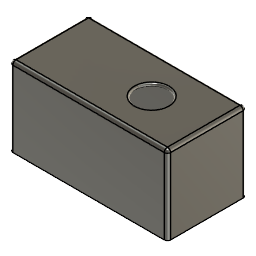
Throttle Box Assembly (Autodesk Fusion 360 archive; units mm, degrees)
design "Cover"
part number: 2026-03-17-12-51-27-306
Autodesk Fusion 360 part; units mm, degrees
sketch "Bottom" plane through (0, 0, 0) normal (0, 0, 1) x (1, 0, 0)
  line L0 (48, 25) -> (-48, 25)
  line L1 (-50, 23) -> (-50, -23)
  line L2 (-48, -25) -> (48, -25)
  line L3 (50, -23) -> (50, 23)
  line L4 (50, 25) -> (-50, -25) construction
  line L5 (-50, 25) -> (50, -25) construction
  arc A0 (-48, 25) -> (-50, 23) centre (-48, 23) ccw
  arc A1 (-50, -23) -> (-48, -25) centre (-48, -23) ccw
  arc A2 (48, -25) -> (50, -23) centre (48, -23) ccw
  arc A3 (50, 23) -> (48, 25) centre (48, 23) ccw
  line L6 (-50, 25) -> (-47, 25)
  line L7 (-47, 25) -> (-47, 22)
  line L8 (-47, 22) -> (-50, 22)
  line L9 (-50, 22) -> (-50, 25)
  circle A4 centre (-47, 22) radius 1.75
  circle A5 centre (-47, 22) radius 3
  line L10 (48, -23) -> (48, 23)
  line L11 (48, 23) -> (-48, 23)
  line L12 (-48, 23) -> (-48, -23)
  line L13 (-48, -23) -> (48, -23)
  circle A6 centre (47, 22) radius 3
  circle A7 centre (47, 22) radius 1.75
  circle A8 centre (-47, -22) radius 3
  circle A9 centre (-47, -22) radius 1.75
  circle A10 centre (47, -22) radius 3
  circle A11 centre (47, -22) radius 1.75
  dimension "d1" = 100
  dimension "d2" = 50
  dimension "d3" = 2
  dimension "d5" = 3
  dimension "d6" = 3
  dimension "d7" = 3.5
  dimension "d8" = 6
  dimension "d23" = -2
  dimension "d62" = 94
  dimension "d63" = -44
  constraint horizontal L0
  constraint perpendicular L0 L1
  constraint parallel L0 L2
  constraint parallel L1 L3
  constraint coincident L4 origin
  constraint coincident L5 origin
  constraint coincident L5.start L0
  constraint coincident L5.start L1
  constraint tangent L0 A0
  constraint tangent L1 A0
  constraint coincident L4.end L1
  constraint coincident L4.end L2
  constraint tangent L1 A1
  constraint tangent L2 A1
  constraint equal A0 A1
  constraint coincident L5.end L2
  constraint coincident L5.end L3
  constraint tangent L2 A2
  constraint tangent L3 A2
  constraint equal A0 A2
  constraint coincident L4.start L3
  constraint coincident L4.start L0
  constraint tangent L3 A3
  constraint tangent L0 A3
  constraint equal A0 A3
  constraint horizontal L6
  constraint vertical L7
  constraint horizontal L8
  constraint vertical L9
  constraint coincident L7.end L8.start
  constraint concentric A4 A5
  measures "d1" distance of L4.end L5.end
  measures "d2" distance of L5.start L4.end
  measures "d3" radius of A0
  measures "d5" distance of L5.start L6.end
  measures "d6" distance of L5.start L8.end
  measures "d7" diameter of A4
  measures "d8" diameter of A5
extrude "Extrude3" add sketch "Bottom" along normal blind 48 contours L0 L1 A0 L6 L9 A5 | L7 A4 A5 L11 | L7 L8 A4 A5 | L0 A5 L11 A6 | L0 L3 A3 A6 | L10 L11 A6 A7 | L1 A5 L12 A8 | L8 A4 A5 L12 | A4 A5 L11 L12 | L3 L10 A6 A10 | L10 L11 A6 A7 | L1 L2 A1 A8 | L12 L13 A8 A9 | L10 L13 A10 A11 | L2 L3 A2 A10 | L12 L13 A8 A9 | L2 L13 A8 A10 | L10 L13 A10 A11
sketch "Top" plane through (0, 0, 48) normal (0, 0, 1) x (-1, 0, 0)
  circle A0 centre (47, 22) radius 1.75
  circle A1 centre (-47, -22) radius 1.75
  circle A2 centre (-47, 22) radius 1.75
  line L0 (48, 19.1716) -> (48, -19.1716)
  arc A3 (48, -19.1716) -> (44.1716, -23) centre (47, -22) ccw
  line L1 (44.1716, -23) -> (-44.1716, -23)
  arc A4 (-44.1716, -23) -> (-48, -19.1716) centre (-47, -22) ccw
  line L2 (-48, -19.1716) -> (-48, 19.1716)
  arc A5 (-48, 19.1716) -> (-44.1716, 23) centre (-47, 22) ccw
  line L3 (-44.1716, 23) -> (44.1716, 23)
  arc A6 (44.1716, 23) -> (48, 19.1716) centre (47, 22) ccw
  circle A7 centre (47, -22) radius 1.75
  arc A8 (50, 23) -> (48, 25) centre (48, 23) ccw
  line L4 (48, 25) -> (-48, 25)
  arc A9 (-48, 25) -> (-50, 23) centre (-48, 23) ccw
  line L5 (-50, 23) -> (-50, -23)
  arc A10 (-50, -23) -> (-48, -25) centre (-48, -23) ccw
  line L6 (-48, -25) -> (48, -25)
  arc A11 (48, -25) -> (50, -23) centre (48, -23) ccw
  line L7 (50, -23) -> (50, 23)
  line L8 (-45, -20) -> (15, -20)
  line L9 (15, -20) -> (15, 20)
  line L10 (15, 20) -> (-45, 20)
  line L11 (-45, 20) -> (-45, -20)
  line L12 (20, -15.6) -> (45, -15.6)
  line L13 (45, -15.6) -> (45, 15.6)
  line L14 (45, 15.6) -> (20, 15.6)
  line L15 (20, 15.6) -> (20, -15.6)
  line L16 (20, -15.6) -> (45, 15.6) construction
  line L17 (45, -15.6) -> (20, 15.6) construction
  line L18 (43, 13.6) -> (22, 13.6)
  line L19 (22, 13.6) -> (22, -13.6)
  line L20 (22, -13.6) -> (43, -13.6)
  line L21 (43, -13.6) -> (43, 13.6)
  circle A12 centre (-15, 0) radius 10
  line L22 (30, -10.6) -> (35, -10.6)
  line L23 (35, -10.6) -> (35, -5.6)
  line L24 (35, -5.6) -> (30, -5.6)
  line L25 (30, -5.6) -> (30, -10.6)
  point P0 (32.5, 0)
  dimension "d68" = 60
  dimension "d69" = 40
  dimension "d70" = 25
  dimension "d71" = 31.2
  dimension "d72" = -2
  dimension "d73" = 20
  dimension "d77" = 5
  dimension "d78" = 5
  constraint horizontal L8
  constraint vertical L9
  constraint horizontal L10
  constraint vertical L11
  constraint horizontal L12
  constraint perpendicular L12 L13
  constraint parallel L12 L14
  constraint parallel L13 L15
  constraint coincident L16 P0
  constraint coincident L17 P0
  constraint horizontal L22
  constraint vertical L23
  constraint horizontal L24
  constraint vertical L25
  measures "d68" distance of L8.start L8.end
  measures "d69" distance of L8.start L10.end
  measures "d70" distance of L13.end L14.end
  measures "d71" distance of L12.end L13.end
  measures "d73" diameter of A12
  measures "d77" distance of L22.start L22.end
  measures "d78" distance of L22.start L24.end
extrude "Extrude8" add sketch "Top" along normal blind 2 contours A0 | A1 | A2 | L0 A3 L1 A4 A5 L3 A6 L8 L9 L10 | A4 A5 L8 L9 L10 L11 | A5 L10 L11 | A4 L8 L11 | A4 L2 A5 L11 | A7 | A8 L4 A9 L5 A10 L6 A11 L7 | L12 L13 L14 L15 | L18 L19 L20 L21 | A12 | L22 L23 L24 L25
fillet "Fillet13" radius 2 8 edges at (50, 0, 50) (49.4142, 24.4142, 50) (0, 25, 50) (-49.4142, 24.4142, 50) (-50, 0, 50) (-49.4142, -24.4142, 50) (0, -25, 50) (49.4142, -24.4142, 50)
extrude "Extrude9" cut sketch "Top" along normal blind 2 contours A12
extrude "Extrude10" add sketch "Top" against normal blind 11.5 contours L22 L23 L24 L25
fillet "Fillet14" radius 2 8 edges at (-30, 8.1, 48) (-30, 5.6, 42.25) (-30, 10.6, 42.25) (-35, 10.6, 42.25) (-35, 5.6, 42.25) (-32.5, 5.6, 48) (-35, 8.1, 48) (-32.5, 10.6, 48)
fillet "Fillet15" radius 1 2 edges at (24.3233, 3.6162, 48) (24.3233, -3.6162, 50)
fillet "Fillet16" radius 1 16 edges at (44.1716, -23, 24) (48, -19.1716, 24) (48, 19.1716, 24) (44.1716, 23, 24) (-44.1716, 23, 24) (-48, 19.1716, 24) (-48, -19.1716, 24) (-44.1716, -23, 24) (-48, 0, 48) (-44.8787, -19.8787, 48) (0, -23, 48) (44.8787, -19.8787, 48) (48, 0, 48) (0, 23, 48) (44.8787, 19.8787, 48) (-44.8787, 19.8787, 48)
equation "d51 = 'Control ESP32: WYGB, WYG, WG, B Curtis: RYBG Bypass: YW F/R: YG, BW'"

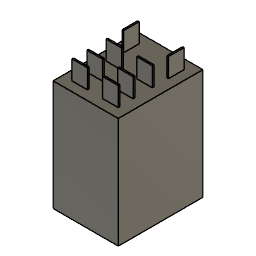
design "YJ2N-LY 24VDC Relay"
part number: 2026-03-24-09-30-35-597
Autodesk Fusion 360 part; units mm, degrees
sketch "Bottom" plane through (0, 0, 0) normal (0, 0, 1) x (1, 0, 0)
  line L0 (10.4, 13.5) -> (-10.4, 13.5)
  line L1 (-10.4, 13.5) -> (-10.4, -13.5)
  line L2 (-10.4, -13.5) -> (10.4, -13.5)
  line L3 (10.4, -13.5) -> (10.4, 13.5)
  line L4 (10.4, 13.5) -> (-10.4, -13.5) construction
  line L5 (-10.4, 13.5) -> (10.4, -13.5) construction
  dimension "d1" = 20.8
  dimension "d2" = 27
  constraint horizontal L0
  constraint perpendicular L0 L1
  constraint parallel L0 L2
  constraint parallel L1 L3
  constraint coincident L4 origin
  constraint coincident L5 origin
  measures "d1" distance of L1.end L2.end
  measures "d2" distance of L0.end L1.end
extrude "Extrude1" add sketch "Bottom" along normal blind 35.25
sketch "Top" plane through (0, 0, 35.25) normal (0, 0, 1) x (-1, 0, 0)
  line L0 (-10.4, 13.5) -> (-10.4, -13.5)
  line L1 (-10.4, -13.5) -> (10.4, -13.5)
  line L2 (10.4, -13.5) -> (10.4, 13.5)
  line L3 (10.4, 13.5) -> (-10.4, 13.5)
  line L4 (-7.4, -10.5) -> (-6.9, -10.5)
  line L5 (-6.9, -10.5) -> (-6.9, -5.5)
  line L6 (-6.9, -5.5) -> (-7.4, -5.5)
  line L7 (-7.4, -5.5) -> (-7.4, -10.5)
  line L8 (6.9, -5.5) -> (6.9, -10.5)
  line L9 (6.9, -10.5) -> (7.4, -10.5)
  line L10 (7.4, -10.5) -> (7.4, -5.5)
  line L11 (7.4, -5.5) -> (6.9, -5.5)
  line L12 (7.4, 10.5) -> (2.4, 10.5)
  line L13 (2.4, 10.5) -> (2.4, 10)
  line L14 (2.4, 10) -> (7.4, 10)
  line L15 (7.4, 10) -> (7.4, 10.5)
  line L16 (-7.4, 10.5) -> (-7.4, 10)
  line L17 (-7.4, 10) -> (-2.4, 10)
  line L18 (-2.4, 10.5) -> (-7.4, 10.5)
  line L19 (-2.4, 10) -> (-2.4, 10.5)
  line L20 (2.4, 5.7) -> (2.4, 5.2)
  line L21 (2.4, 5.2) -> (7.4, 5.2)
  line L22 (7.4, 5.7) -> (2.4, 5.7)
  line L23 (7.4, 5.2) -> (7.4, 5.7)
  line L24 (-7.4, 5.7) -> (-7.4, 5.2)
  line L25 (-7.4, 5.2) -> (-2.4, 5.2)
  line L26 (-2.4, 5.7) -> (-7.4, 5.7)
  line L27 (-2.4, 5.2) -> (-2.4, 5.7)
  line L28 (-7.4, -0.9) -> (-2.4, -0.9)
  line L29 (-7.4, -0.4) -> (-7.4, -0.9)
  line L30 (-2.4, -0.9) -> (-2.4, -0.4)
  line L31 (2.4, -0.4) -> (2.4, -0.9)
  line L32 (2.4, -0.9) -> (7.4, -0.9)
  line L33 (7.4, -0.4) -> (2.4, -0.4)
  line L34 (-2.4, -0.4) -> (-7.4, -0.4)
  line L35 (7.4, -0.9) -> (7.4, -0.4)
  dimension "d7" = 0.5
  dimension "d8" = 5
  dimension "d11" = 14.3
  dimension "d12" = 0
  dimension "d15" = 5
  dimension "d16" = 0.5
  dimension "d19" = -9.8
  dimension "d20" = -4.8
  dimension "d23" = 0
  dimension "d24" = -6.1
  constraint horizontal L4
  constraint vertical L5
  constraint horizontal L6
  constraint vertical L7
  constraint horizontal L12
  constraint vertical L13
  constraint horizontal L14
  constraint vertical L15
  measures "d7" distance of L4.start L4.end
  measures "d8" distance of L4.start L6.end
  measures "d15" distance of L12.start L12.end
  measures "d16" distance of L12.start L14.end
extrude "Extrude2" add sketch "Top" along normal blind 6.1 contours L4 L5 L6 L7 | L8 L9 L10 L11 | L12 L13 L14 L15 | L16 L17 L18 L19 | L20 L21 L22 L23 | L24 L25 L26 L27 | L28 L29 L30 L34 | L31 L32 L33 L35

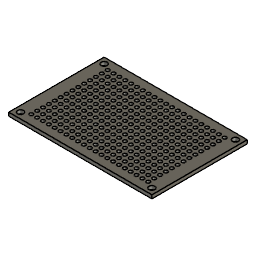
design "Perfboard"
part number: 2026-02-25-23-39-29-210
Autodesk Fusion 360 part; units mm, degrees
sketch "Bottom" plane through (0, 0, 0) normal (0, 0, 1) x (1, 0, 0)
  line L0 (30, 20) -> (-30, 20)
  line L1 (-30, 20) -> (-30, -20)
  line L2 (-30, -20) -> (30, -20)
  line L3 (30, -20) -> (30, 20)
  line L4 (30, 20) -> (-30, -20) construction
  line L5 (-30, 20) -> (30, -20) construction
  circle A0 centre (-27.5, 17.5) radius 1.25
  circle A1 centre (27.5, 17.5) radius 1.25
  circle A2 centre (-27.5, -17.5) radius 1.25
  circle A3 centre (27.5, -17.5) radius 1.25
  circle A4 centre (-24.5, 16) radius 0.75
  circle A5 centre (-22.05, 16) radius 0.75
  circle A6 centre (-19.6, 16) radius 0.75
  circle A7 centre (-17.15, 16) radius 0.75
  circle A8 centre (-14.7, 16) radius 0.75
  circle A9 centre (-12.25, 16) radius 0.75
  circle A10 centre (-9.8, 16) radius 0.75
  circle A11 centre (-7.35, 16) radius 0.75
  circle A12 centre (-4.9, 16) radius 0.75
  circle A13 centre (-2.45, 16) radius 0.75
  circle A14 centre (0, 16) radius 0.75
  circle A15 centre (2.45, 16) radius 0.75
  circle A16 centre (4.9, 16) radius 0.75
  circle A17 centre (7.35, 16) radius 0.75
  circle A18 centre (9.8, 16) radius 0.75
  circle A19 centre (12.25, 16) radius 0.75
  circle A20 centre (14.7, 16) radius 0.75
  circle A21 centre (17.15, 16) radius 0.75
  circle A22 centre (19.6, 16) radius 0.75
  circle A23 centre (22.05, 16) radius 0.75
  circle A24 centre (24.5, 16) radius 0.75
  circle A25 centre (-24.5, 13.5385) radius 0.75
  circle A26 centre (-22.05, 13.5385) radius 0.75
  circle A27 centre (-19.6, 13.5385) radius 0.75
  circle A28 centre (-17.15, 13.5385) radius 0.75
  circle A29 centre (-14.7, 13.5385) radius 0.75
  circle A30 centre (-12.25, 13.5385) radius 0.75
  circle A31 centre (-9.8, 13.5385) radius 0.75
  circle A32 centre (-7.35, 13.5385) radius 0.75
  circle A33 centre (-4.9, 13.5385) radius 0.75
  circle A34 centre (-2.45, 13.5385) radius 0.75
  circle A35 centre (0, 13.5385) radius 0.75
  circle A36 centre (2.45, 13.5385) radius 0.75
  circle A37 centre (4.9, 13.5385) radius 0.75
  circle A38 centre (7.35, 13.5385) radius 0.75
  circle A39 centre (9.8, 13.5385) radius 0.75
  circle A40 centre (12.25, 13.5385) radius 0.75
  circle A41 centre (14.7, 13.5385) radius 0.75
  circle A42 centre (17.15, 13.5385) radius 0.75
  circle A43 centre (19.6, 13.5385) radius 0.75
  circle A44 centre (22.05, 13.5385) radius 0.75
  circle A45 centre (24.5, 13.5385) radius 0.75
  circle A46 centre (-24.5, 11.0769) radius 0.75
  circle A47 centre (-22.05, 11.0769) radius 0.75
  circle A48 centre (-19.6, 11.0769) radius 0.75
  circle A49 centre (-17.15, 11.0769) radius 0.75
  circle A50 centre (-14.7, 11.0769) radius 0.75
  circle A51 centre (-12.25, 11.0769) radius 0.75
  circle A52 centre (-9.8, 11.0769) radius 0.75
  circle A53 centre (-7.35, 11.0769) radius 0.75
  circle A54 centre (-4.9, 11.0769) radius 0.75
  circle A55 centre (-2.45, 11.0769) radius 0.75
  circle A56 centre (0, 11.0769) radius 0.75
  circle A57 centre (2.45, 11.0769) radius 0.75
  circle A58 centre (4.9, 11.0769) radius 0.75
  circle A59 centre (7.35, 11.0769) radius 0.75
  circle A60 centre (9.8, 11.0769) radius 0.75
  circle A61 centre (12.25, 11.0769) radius 0.75
  circle A62 centre (14.7, 11.0769) radius 0.75
  circle A63 centre (17.15, 11.0769) radius 0.75
  circle A64 centre (19.6, 11.0769) radius 0.75
  circle A65 centre (22.05, 11.0769) radius 0.75
  circle A66 centre (24.5, 11.0769) radius 0.75
  circle A67 centre (-24.5, 8.6154) radius 0.75
  circle A68 centre (-22.05, 8.6154) radius 0.75
  circle A69 centre (-19.6, 8.6154) radius 0.75
  circle A70 centre (-17.15, 8.6154) radius 0.75
  circle A71 centre (-14.7, 8.6154) radius 0.75
  circle A72 centre (-12.25, 8.6154) radius 0.75
  circle A73 centre (-9.8, 8.6154) radius 0.75
  circle A74 centre (-7.35, 8.6154) radius 0.75
  circle A75 centre (-4.9, 8.6154) radius 0.75
  circle A76 centre (-2.45, 8.6154) radius 0.75
  circle A77 centre (0, 8.6154) radius 0.75
  circle A78 centre (2.45, 8.6154) radius 0.75
  circle A79 centre (4.9, 8.6154) radius 0.75
  circle A80 centre (7.35, 8.6154) radius 0.75
  circle A81 centre (9.8, 8.6154) radius 0.75
  circle A82 centre (12.25, 8.6154) radius 0.75
  circle A83 centre (14.7, 8.6154) radius 0.75
  circle A84 centre (17.15, 8.6154) radius 0.75
  circle A85 centre (19.6, 8.6154) radius 0.75
  circle A86 centre (22.05, 8.6154) radius 0.75
  circle A87 centre (24.5, 8.6154) radius 0.75
  circle A88 centre (-24.5, 6.1538) radius 0.75
  circle A89 centre (-22.05, 6.1538) radius 0.75
  circle A90 centre (-19.6, 6.1538) radius 0.75
  circle A91 centre (-17.15, 6.1538) radius 0.75
  circle A92 centre (-14.7, 6.1538) radius 0.75
  circle A93 centre (-12.25, 6.1538) radius 0.75
  circle A94 centre (-9.8, 6.1538) radius 0.75
  circle A95 centre (-7.35, 6.1538) radius 0.75
  circle A96 centre (-4.9, 6.1538) radius 0.75
  circle A97 centre (-2.45, 6.1538) radius 0.75
  circle A98 centre (0, 6.1538) radius 0.75
  circle A99 centre (2.45, 6.1538) radius 0.75
  circle A100 centre (4.9, 6.1538) radius 0.75
  circle A101 centre (7.35, 6.1538) radius 0.75
  circle A102 centre (9.8, 6.1538) radius 0.75
  circle A103 centre (12.25, 6.1538) radius 0.75
  circle A104 centre (14.7, 6.1538) radius 0.75
  circle A105 centre (17.15, 6.1538) radius 0.75
  circle A106 centre (19.6, 6.1538) radius 0.75
  circle A107 centre (22.05, 6.1538) radius 0.75
  circle A108 centre (24.5, 6.1538) radius 0.75
  circle A109 centre (-24.5, 3.6923) radius 0.75
  circle A110 centre (-22.05, 3.6923) radius 0.75
  circle A111 centre (-19.6, 3.6923) radius 0.75
  circle A112 centre (-17.15, 3.6923) radius 0.75
  circle A113 centre (-14.7, 3.6923) radius 0.75
  circle A114 centre (-12.25, 3.6923) radius 0.75
  circle A115 centre (-9.8, 3.6923) radius 0.75
  circle A116 centre (-7.35, 3.6923) radius 0.75
  circle A117 centre (-4.9, 3.6923) radius 0.75
  circle A118 centre (-2.45, 3.6923) radius 0.75
  circle A119 centre (0, 3.6923) radius 0.75
  circle A120 centre (2.45, 3.6923) radius 0.75
  circle A121 centre (4.9, 3.6923) radius 0.75
  circle A122 centre (7.35, 3.6923) radius 0.75
  circle A123 centre (9.8, 3.6923) radius 0.75
  circle A124 centre (12.25, 3.6923) radius 0.75
  circle A125 centre (14.7, 3.6923) radius 0.75
  circle A126 centre (17.15, 3.6923) radius 0.75
  circle A127 centre (19.6, 3.6923) radius 0.75
  circle A128 centre (22.05, 3.6923) radius 0.75
  circle A129 centre (24.5, 3.6923) radius 0.75
  circle A130 centre (-24.5, 1.2308) radius 0.75
  circle A131 centre (-22.05, 1.2308) radius 0.75
  circle A132 centre (-19.6, 1.2308) radius 0.75
  circle A133 centre (-17.15, 1.2308) radius 0.75
  circle A134 centre (-14.7, 1.2308) radius 0.75
  circle A135 centre (-12.25, 1.2308) radius 0.75
  circle A136 centre (-9.8, 1.2308) radius 0.75
  circle A137 centre (-7.35, 1.2308) radius 0.75
  circle A138 centre (-4.9, 1.2308) radius 0.75
  circle A139 centre (-2.45, 1.2308) radius 0.75
  circle A140 centre (0, 1.2308) radius 0.75
  circle A141 centre (2.45, 1.2308) radius 0.75
  circle A142 centre (4.9, 1.2308) radius 0.75
  circle A143 centre (7.35, 1.2308) radius 0.75
  circle A144 centre (9.8, 1.2308) radius 0.75
  circle A145 centre (12.25, 1.2308) radius 0.75
  circle A146 centre (14.7, 1.2308) radius 0.75
  circle A147 centre (17.15, 1.2308) radius 0.75
  circle A148 centre (19.6, 1.2308) radius 0.75
  circle A149 centre (22.05, 1.2308) radius 0.75
  circle A150 centre (24.5, 1.2308) radius 0.75
  circle A151 centre (-24.5, -1.2308) radius 0.75
  circle A152 centre (-22.05, -1.2308) radius 0.75
  circle A153 centre (-19.6, -1.2308) radius 0.75
  circle A154 centre (-17.15, -1.2308) radius 0.75
  circle A155 centre (-14.7, -1.2308) radius 0.75
  circle A156 centre (-12.25, -1.2308) radius 0.75
  circle A157 centre (-9.8, -1.2308) radius 0.75
  circle A158 centre (-7.35, -1.2308) radius 0.75
  circle A159 centre (-4.9, -1.2308) radius 0.75
  circle A160 centre (-2.45, -1.2308) radius 0.75
  circle A161 centre (0, -1.2308) radius 0.75
  circle A162 centre (2.45, -1.2308) radius 0.75
  circle A163 centre (4.9, -1.2308) radius 0.75
  circle A164 centre (7.35, -1.2308) radius 0.75
  circle A165 centre (9.8, -1.2308) radius 0.75
  circle A166 centre (12.25, -1.2308) radius 0.75
  circle A167 centre (14.7, -1.2308) radius 0.75
  circle A168 centre (17.15, -1.2308) radius 0.75
  circle A169 centre (19.6, -1.2308) radius 0.75
  circle A170 centre (22.05, -1.2308) radius 0.75
  circle A171 centre (24.5, -1.2308) radius 0.75
  circle A172 centre (-24.5, -3.6923) radius 0.75
  circle A173 centre (-22.05, -3.6923) radius 0.75
  circle A174 centre (-19.6, -3.6923) radius 0.75
  circle A175 centre (-17.15, -3.6923) radius 0.75
  circle A176 centre (-14.7, -3.6923) radius 0.75
  circle A177 centre (-12.25, -3.6923) radius 0.75
  circle A178 centre (-9.8, -3.6923) radius 0.75
  circle A179 centre (-7.35, -3.6923) radius 0.75
  circle A180 centre (-4.9, -3.6923) radius 0.75
  circle A181 centre (-2.45, -3.6923) radius 0.75
  circle A182 centre (0, -3.6923) radius 0.75
  circle A183 centre (2.45, -3.6923) radius 0.75
  circle A184 centre (4.9, -3.6923) radius 0.75
  circle A185 centre (7.35, -3.6923) radius 0.75
  circle A186 centre (9.8, -3.6923) radius 0.75
  circle A187 centre (12.25, -3.6923) radius 0.75
  circle A188 centre (14.7, -3.6923) radius 0.75
  circle A189 centre (17.15, -3.6923) radius 0.75
  circle A190 centre (19.6, -3.6923) radius 0.75
  circle A191 centre (22.05, -3.6923) radius 0.75
  circle A192 centre (24.5, -3.6923) radius 0.75
  circle A193 centre (-24.5, -6.1538) radius 0.75
  circle A194 centre (-22.05, -6.1538) radius 0.75
  circle A195 centre (-19.6, -6.1538) radius 0.75
  circle A196 centre (-17.15, -6.1538) radius 0.75
  circle A197 centre (-14.7, -6.1538) radius 0.75
  circle A198 centre (-12.25, -6.1538) radius 0.75
  circle A199 centre (-9.8, -6.1538) radius 0.75
  circle A200 centre (-7.35, -6.1538) radius 0.75
  circle A201 centre (-4.9, -6.1538) radius 0.75
  circle A202 centre (-2.45, -6.1538) radius 0.75
  circle A203 centre (0, -6.1538) radius 0.75
  circle A204 centre (2.45, -6.1538) radius 0.75
  circle A205 centre (4.9, -6.1538) radius 0.75
  circle A206 centre (7.35, -6.1538) radius 0.75
  circle A207 centre (9.8, -6.1538) radius 0.75
  circle A208 centre (12.25, -6.1538) radius 0.75
  circle A209 centre (14.7, -6.1538) radius 0.75
  circle A210 centre (17.15, -6.1538) radius 0.75
  circle A211 centre (19.6, -6.1538) radius 0.75
  circle A212 centre (22.05, -6.1538) radius 0.75
  circle A213 centre (24.5, -6.1538) radius 0.75
  circle A214 centre (-24.5, -8.6154) radius 0.75
  circle A215 centre (-22.05, -8.6154) radius 0.75
  circle A216 centre (-19.6, -8.6154) radius 0.75
  circle A217 centre (-17.15, -8.6154) radius 0.75
  circle A218 centre (-14.7, -8.6154) radius 0.75
  circle A219 centre (-12.25, -8.6154) radius 0.75
  circle A220 centre (-9.8, -8.6154) radius 0.75
  circle A221 centre (-7.35, -8.6154) radius 0.75
  circle A222 centre (-4.9, -8.6154) radius 0.75
  circle A223 centre (-2.45, -8.6154) radius 0.75
  circle A224 centre (0, -8.6154) radius 0.75
  circle A225 centre (2.45, -8.6154) radius 0.75
  circle A226 centre (4.9, -8.6154) radius 0.75
  circle A227 centre (7.35, -8.6154) radius 0.75
  circle A228 centre (9.8, -8.6154) radius 0.75
  circle A229 centre (12.25, -8.6154) radius 0.75
  circle A230 centre (14.7, -8.6154) radius 0.75
  circle A231 centre (17.15, -8.6154) radius 0.75
  circle A232 centre (19.6, -8.6154) radius 0.75
  circle A233 centre (22.05, -8.6154) radius 0.75
  circle A234 centre (24.5, -8.6154) radius 0.75
  circle A235 centre (-24.5, -11.0769) radius 0.75
  circle A236 centre (-22.05, -11.0769) radius 0.75
  circle A237 centre (-19.6, -11.0769) radius 0.75
  circle A238 centre (-17.15, -11.0769) radius 0.75
  circle A239 centre (-14.7, -11.0769) radius 0.75
  circle A240 centre (-12.25, -11.0769) radius 0.75
  circle A241 centre (-9.8, -11.0769) radius 0.75
  circle A242 centre (-7.35, -11.0769) radius 0.75
  circle A243 centre (-4.9, -11.0769) radius 0.75
  circle A244 centre (-2.45, -11.0769) radius 0.75
  circle A245 centre (0, -11.0769) radius 0.75
  circle A246 centre (2.45, -11.0769) radius 0.75
  circle A247 centre (4.9, -11.0769) radius 0.75
  circle A248 centre (7.35, -11.0769) radius 0.75
  circle A249 centre (9.8, -11.0769) radius 0.75
  circle A250 centre (12.25, -11.0769) radius 0.75
  circle A251 centre (14.7, -11.0769) radius 0.75
  circle A252 centre (17.15, -11.0769) radius 0.75
  circle A253 centre (19.6, -11.0769) radius 0.75
  circle A254 centre (22.05, -11.0769) radius 0.75
  circle A255 centre (24.5, -11.0769) radius 0.75
  circle A256 centre (-24.5, -13.5385) radius 0.75
  circle A257 centre (-22.05, -13.5385) radius 0.75
  circle A258 centre (-19.6, -13.5385) radius 0.75
  circle A259 centre (-17.15, -13.5385) radius 0.75
  circle A260 centre (-14.7, -13.5385) radius 0.75
  circle A261 centre (-12.25, -13.5385) radius 0.75
  circle A262 centre (-9.8, -13.5385) radius 0.75
  circle A263 centre (-7.35, -13.5385) radius 0.75
  circle A264 centre (-4.9, -13.5385) radius 0.75
  circle A265 centre (-2.45, -13.5385) radius 0.75
  circle A266 centre (0, -13.5385) radius 0.75
  circle A267 centre (2.45, -13.5385) radius 0.75
  circle A268 centre (4.9, -13.5385) radius 0.75
  circle A269 centre (7.35, -13.5385) radius 0.75
  circle A270 centre (9.8, -13.5385) radius 0.75
  circle A271 centre (12.25, -13.5385) radius 0.75
  circle A272 centre (14.7, -13.5385) radius 0.75
  circle A273 centre (17.15, -13.5385) radius 0.75
  circle A274 centre (19.6, -13.5385) radius 0.75
  circle A275 centre (22.05, -13.5385) radius 0.75
  circle A276 centre (24.5, -13.5385) radius 0.75
  circle A277 centre (-24.5, -16) radius 0.75
  circle A278 centre (-22.05, -16) radius 0.75
  circle A279 centre (-19.6, -16) radius 0.75
  circle A280 centre (-17.15, -16) radius 0.75
  circle A281 centre (-14.7, -16) radius 0.75
  circle A282 centre (-12.25, -16) radius 0.75
  circle A283 centre (-9.8, -16) radius 0.75
  circle A284 centre (-7.35, -16) radius 0.75
  circle A285 centre (-4.9, -16) radius 0.75
  circle A286 centre (-2.45, -16) radius 0.75
  circle A287 centre (0, -16) radius 0.75
  circle A288 centre (2.45, -16) radius 0.75
  circle A289 centre (4.9, -16) radius 0.75
  circle A290 centre (7.35, -16) radius 0.75
  circle A291 centre (9.8, -16) radius 0.75
  circle A292 centre (12.25, -16) radius 0.75
  circle A293 centre (14.7, -16) radius 0.75
  circle A294 centre (17.15, -16) radius 0.75
  circle A295 centre (19.6, -16) radius 0.75
  circle A296 centre (22.05, -16) radius 0.75
  circle A297 centre (24.5, -16) radius 0.75
  dimension "d1" = 60
  dimension "d2" = 2.5
  dimension "d5" = 55
  dimension "d6" = -35
  dimension "d7" = 1.5
  dimension "d10" = 49
  dimension "d11" = -32
  constraint horizontal L0
  constraint perpendicular L0 L1
  constraint parallel L0 L2
  constraint parallel L1 L3
  constraint coincident L4 origin
  constraint coincident L5 origin
  measures "d1" distance of L1.end L2.end
  measures "d2" diameter of A0
  measures "d7" diameter of A4
extrude "Extrude1" add sketch "Bottom" along normal blind 1.5

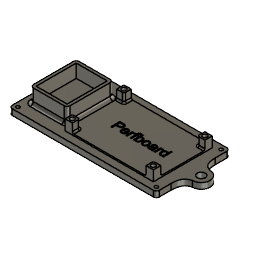
design "Mount"
part number: 2026-02-23-15-20-57-975
Autodesk Fusion 360 part; units mm, degrees
sketch "Bottom" plane through (0, 0, 0) normal (0, 0, 1) x (1, 0, 0)
  line L0 (50, 25) -> (-50, 25)
  line L1 (-50, 25) -> (-50, -25)
  line L2 (-50, -25) -> (50, -25)
  line L3 (50, -25) -> (50, 25)
  line L4 (50, 25) -> (-50, -25) construction
  line L5 (-50, 25) -> (50, -25) construction
  spline S0 degree 5 poles (50, -15) (50.0023, -14.6955) (50.016, -14.097) (50.0639, -13.2309) (50.1832, -12.1401) (50.4313, -10.8912) (50.7883, -9.768) (51.2646, -8.7828) (51.8686, -7.9453) (52.5996, -7.2545) (53.4497, -6.7014) (54.2182, -6.3612) (54.8412, -6.1599) (55.277, -6.0494) (55.5, -6) knots 0 0 0 0 0 0 0.1 0.2 0.3 0.4 0.5 0.6 0.7 0.8 0.9 1 1 1 1 1 1
  circle A0 centre (55.5, 0) radius 6
  circle A1 centre (55.5, 0) radius 2.75
  circle A2 centre (55.5, 0) radius 5
  line L6 (50, 0) -> (55.5, 0)
  spline S1 degree 5 poles (50, 15) (50.0023, 14.6955) (50.016, 14.097) (50.0639, 13.2309) (50.1832, 12.1401) (50.4313, 10.8912) (50.7883, 9.768) (51.2646, 8.7828) (51.8686, 7.9453) (52.5996, 7.2545) (53.4497, 6.7014) (54.2182, 6.3612) (54.8412, 6.1599) (55.277, 6.0494) (55.5, 6) knots 0 0 0 0 0 0 0.1 0.2 0.3 0.4 0.5 0.6 0.7 0.8 0.9 1 1 1 1 1 1
  circle A3 centre (-47, 22) radius 1.15
  circle A4 centre (-47, 22) radius 2
  circle A5 centre (47, 22) radius 1.15
  circle A6 centre (47, 22) radius 2
  circle A7 centre (-47, -22) radius 1.15
  circle A8 centre (-47, -22) radius 2
  circle A9 centre (47, -22) radius 1.15
  circle A10 centre (47, -22) radius 2
  point P0 (51.5, -8.5)
  point P1 (51.5, 8.5)
  dimension "d1" = 100
  dimension "d2" = 50
  dimension "d329" = 5.5
  dimension "d330" = 5.5
  dimension "d331" = 12
  dimension "d332" = 10
  dimension "d518" = 2.3
  dimension "d519" = 4
  dimension "d530" = 94
  dimension "d531" = -44
  constraint horizontal L0
  constraint perpendicular L0 L1
  constraint parallel L0 L2
  constraint parallel L1 L3
  constraint coincident L4 origin
  constraint coincident L5 origin
  constraint coincident A0.centre A1.centre
  constraint concentric A0 A1
  constraint coincident S1.end A0
  constraint coincident S0.end A0
  constraint concentric A3 A4
  measures "d1" distance of L1.end L2.end
  measures "d2" distance of L0.end L1.end
  measures "d329" distance of A0.centre L6.start
  measures "d330" diameter of A1
  measures "d331" diameter of A0
  measures "d332" diameter of A2
  measures "d518" diameter of A3
  measures "d519" diameter of A4
extrude "Extrude40" add sketch "Bottom" along normal blind 4 contours L0 L1 L2 L3 A0 | L3 A0 S1 | L3 A0 | L3 A0 | L3 S0 A0 | A3 | A4 | A5 | A6 | A7 | A8 | A9 | A10
sketch "Mounting Area" plane through (0, 0, 4) normal (0, 0, 1) x (-1, 0, 0)
  line L0 (-43, -20) -> (17, -20)
  line L1 (17, -20) -> (17, 20)
  line L2 (17, 20) -> (-43, 20)
  line L3 (-43, 20) -> (-43, -20)
  line L4 (22, -13.6) -> (43, -13.6)
  line L5 (43, -13.6) -> (43, 13.6)
  line L6 (43, 13.6) -> (22, 13.6)
  line L7 (22, 13.6) -> (22, -13.6)
  line L8 (22, -13.6) -> (43, 13.6) construction
  line L9 (43, -13.6) -> (22, 13.6) construction
  line L10 (45, 15.6) -> (20, 15.6)
  line L11 (20, 15.6) -> (20, -15.6)
  line L12 (20, -15.6) -> (45, -15.6)
  line L13 (45, -15.6) -> (45, 15.6)
  point P0 (32.5, 0)
  dimension "d532" = 60
  dimension "d533" = 40
  dimension "d534" = 21
  dimension "d535" = 27.2
  dimension "d536" = 2
  constraint horizontal L0
  constraint vertical L1
  constraint horizontal L2
  constraint vertical L3
  constraint horizontal L4
  constraint perpendicular L4 L5
  constraint parallel L4 L6
  constraint parallel L5 L7
  constraint coincident L8 P0
  constraint coincident L9 P0
  measures "d532" distance of L0.start L0.end
  measures "d533" distance of L0.start L2.end
  measures "d534" distance of L5.end L6.end
  measures "d535" distance of L4.end L5.end
extrude "Extrude72" add sketch "Mounting Area" along normal blind 1 contours L0 L1 L2 L3 | L4 L5 L6 L7
extrude "Extrude73" add sketch "Mounting Area" along normal blind 10 contours L10 L11 L12 L13
extrude "Extrude74" add sketch "Bottom" along normal blind 4 contours A2
extrude "Extrude75" cut sketch "Bottom" along normal blind 8 contours A3 | A5 | A7 | A9
extrude "Extrude76" cut sketch "Bottom" along normal blind 2 contours A4 | A6 | A8 | A10
fillet "Fillet42" radius 2 4 edges at (50, -25, 2) (50, 25, 2) (-50, -25, 2) (-50, 25, 2)
fillet "Fillet43" radius 2 8 edges at (-20, -15.6, 9) (-45, -15.6, 9) (-45, 15.6, 9) (-20, 15.6, 9) (-20, 0, 4) (-32.5, 15.6, 4) (-45, 0, 4) (-32.5, -15.6, 4)
sketch "Perfboard Mount" plane through (0, 0, 5) normal (0, 0, 1) x (-1, 0, 0)
  line L0 (-43, 20) -> (-43, -20)
  line L1 (-43, -20) -> (17, -20)
  line L2 (17, -20) -> (17, 20)
  line L3 (17, 20) -> (-43, 20)
  line L4 (-43, 20) -> (-38, 20)
  line L5 (-38, 20) -> (-38, 15)
  line L6 (-38, 15) -> (-43, 15)
  line L7 (-43, 15) -> (-43, 20)
  circle A0 centre (-40.5, 17.5) radius 1.5
  line L8 (17, 15) -> (12, 15)
  line L9 (12, 15) -> (12, 20)
  circle A1 centre (14.5, 17.5) radius 1.5
  line L10 (17, 20) -> (17, 15)
  line L11 (12, 20) -> (17, 20)
  line L12 (-38, -20) -> (-43, -20)
  line L13 (-43, -20) -> (-43, -15)
  circle A2 centre (-40.5, -17.5) radius 1.5
  line L14 (-38, -15) -> (-38, -20)
  line L15 (-43, -15) -> (-38, -15)
  line L16 (17, -20) -> (12, -20)
  line L17 (12, -20) -> (12, -15)
  circle A3 centre (14.5, -17.5) radius 1.5
  line L18 (17, -15) -> (17, -20)
  line L19 (12, -15) -> (17, -15)
  line L20 (5, 15) -> (-35, 15) construction
  line L21 (-35, 15) -> (-35, -15) construction
  line L22 (-35, -15) -> (5, -15) construction
  line L23 (5, -15) -> (5, 15) construction
  dimension "d551" = 5
  dimension "d552" = 5
  dimension "d553" = 3
  dimension "d556" = 55
  dimension "d557" = -35
  dimension "d558" = 6
  text T0 "Perfboard" font "Arial" height 6 align centre middle in box 40 x 30 at (5, 15) x (-1, 0) y (0, -1) spacing 1 kerned
  constraint horizontal L4
  constraint vertical L5
  constraint horizontal L6
  constraint vertical L7
  constraint coincident L0.start L3.end
  measures "d551" distance of L0.start L4.end
  measures "d552" distance of L0.start L6.end
  measures "d553" diameter of A0
extrude "Extrude77" add sketch "Perfboard Mount" along normal blind 6 contours L0 L3 L4 L5 L6 L7 | L0 L1 L12 L13 L14 L15 | L2 L3 L8 L9 L10 L11 | L1 L2 L16 L17 L18 L19
extrude "Extrude78" cut sketch "Perfboard Mount" against normal blind 1 text T0
fillet "Fillet44" radius 1 12 edges at (-12, 15, 8) (-12, 17.5, 5) (-14.5, 15, 5) (-12, -17.5, 5) (-12, -15, 8) (-14.5, -15, 5) (40.5, -15, 5) (38, -15, 8) (38, -17.5, 5) (40.5, 15, 5) (38, 17.5, 5) (38, 15, 8)
equation "d559 = 'Perfboard'"
equation "d314 = '5V Relay'"
